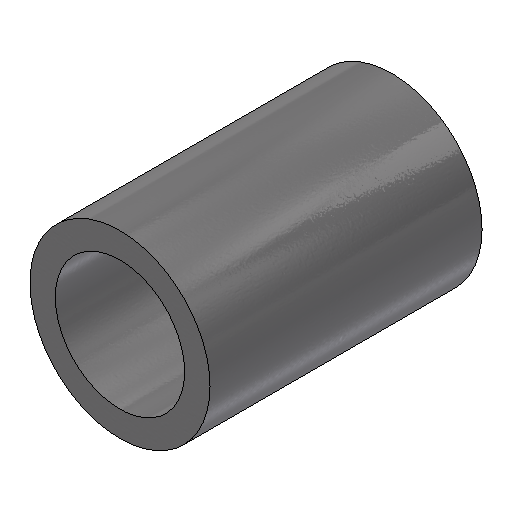
# Autodesk Inventor part: TL20240701-10110CV-008
Saved by Autodesk Inventor 2022.5 (Build 265521000, 521)
## iProperties
Category: DRIVE UNIT ASSY
Manager: 호상태
Company: 현대 트랜시스(대유)
Created: 2023-01-20
Part Number: TL20240701-10110CV-008
Project: SW PJT
Checked By: 김형민
Engr Approved By: 김시현
Material: S45C
Description: 0
Document SubType Name: Modeling
Mfg Approved By: 호상태
Designer: 박성규
Density: 7.87 g/cm^3
Appearance: Plating Zinc White
Stock Number: 008
User Status: 1 x18
DETAIL: Coveryor Assembly
M/C TITLE: MEa/NEa차종 시트조립라인
SPECIFICATION: TL20221201-000000CV-011
DocNumber: 221118_Standard_v1
Folder: .\
VDS_Category: 엔지니어링
Detail Description: Processed products
Title: COLLAR
Subject: SW차종 시트조립라인
Author: 박성규
Revision Number: A
Autodesk Inventor part; units mm, degrees
ref_plane "YZ Plane" through (0, 0, 0) normal (1, 0, 0) x (0, 1, 0)
ref_plane "XZ Plane" through (0, 0, 0) normal (0, 1, 0) x (-1, 0, 0)
ref_plane "XY Plane" through (0, 0, 0) normal (0, 0, 1) x (1, 0, 0)
sketch "스케치10" plane through (0, 0, 0) normal (0, 0, 1) x (1, 0, 0)
  circle A0 centre (0, 0) radius 14
  circle A1 centre (0, 0) radius 10.05
  dimension "d57" = 28
  dimension "d58" = 20.1
  constraints: 2 centre point, 2 coincident
  measures "d57" diameter of A0
  measures "d58" diameter of A1
extrude "돌출4" add sketch "스케치10" along normal blind 42.3
